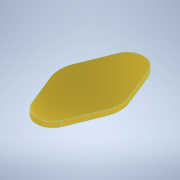
# Autodesk Inventor part: Diamond-Box-Lid
Saved by Autodesk Inventor 2022.4 (Build 264492000, 492)
## iProperties
Created: 2024-02-29
Part Number: Diamond-Box-Lid
Material: Generic
Document SubType Name: Modeling
Designer: t60147996
Density: 1 g/cm^3
Appearance: Sky Blue Dark
Author: t60147996
Autodesk Inventor part; units mm, degrees
ref_plane "YZ Plane" through (0, 0, 0) normal (1, 0, 0) x (0, 1, 0)
ref_plane "XZ Plane" through (0, 0, 0) normal (0, 1, 0) x (-1, 0, 0)
ref_plane "XY Plane" through (0, 0, 0) normal (0, 0, 1) x (1, 0, 0)
sketch "Sketch1" plane through (0, 0, 0) normal (0, 1, 0) x (-1, 0, 0)
  circle A0 centre (0, 0) radius 41.275
  circle A1 centre (0, 50.8) radius 22.225
  circle A2 centre (0, -50.8) radius 22.225
  line L0 (38.2629, 15.4781) -> (20.6031, 59.1344)
  line L1 (-38.2629, 15.4781) -> (-20.6031, 59.1344)
  line L2 (-38.2629, -15.4781) -> (-20.6031, -59.1344)
  line L3 (38.2629, -15.4781) -> (20.6031, -59.1344)
  dimension "d0" = 82.55
  dimension "d1" = 44.45
  dimension "d2" = 44.45
  dimension "d3" = 50.8
  dimension "d4" = 50.8
  constraints: 8 end point, 8 point on circle, 8 tangent, 3 centre point, 2 vertical alignment, 1 coincident
  measures "d0" diameter of A0
  measures "d1" diameter of A1
  measures "d2" diameter of A2
  measures "d3" distance of point (0, 0) A1.centre
  measures "d4" distance of point (0, 0) A2.centre
extrude "Extrusion1" add sketch "Sketch1" along normal blind 7.62
shell "Shell2" thickness 2.54 removed faces 1 at (-6.8677, 0, -30.0302)
body "Solid1"
